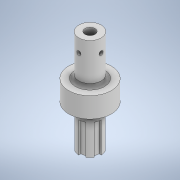
# Autodesk Inventor part: shaft
Saved by Autodesk Inventor 2020.3 (Build 243373000, 373)
## iProperties
Created: 2020-08-08
Part Number: shaft
Material: Generic
Document SubType Name: Modeling
Designer: joesp
Density: 1 g/cm^3
Appearance: Default
Author: joesp
Autodesk Inventor part; units mm, degrees
ref_plane "YZ Plane" through (0, 0, 0) normal (1, 0, 0) x (0, 1, 0)
ref_plane "XZ Plane" through (0, 0, 0) normal (0, 1, 0) x (-1, 0, 0)
ref_plane "XY Plane" through (0, 0, 0) normal (0, 0, 1) x (1, 0, 0)
sketch "Sketch1" plane through (0, 0, 0) normal (1, 0, 0) x (0, 1, 0)
  line L0 (0, 0) -> (100, 0)
  line L1 (100, 0) -> (100, -11)
  line L2 (100, -11) -> (0, -11)
  line L3 (0, -11) -> (0, 0)
  line L4 (60, -11) -> (40, -11)
  line L5 (40, -11) -> (40, -21)
  line L6 (40, -21) -> (60, -21)
  line L7 (60, -21) -> (60, -11)
  line L8 (0, -11) -> (100, -11)
  line L9 (100, -11) -> (100, -5)
  line L10 (100, -5) -> (0, -5)
  line L11 (0, -5) -> (0, -11)
  circle A0 centre (39, -12) radius 2.5
  line L12 (37.2322, -10.2322) -> (40.7678, -13.7678) construction
  circle A1 centre (61, -12) radius 2.5
  line L13 (62.7678, -10.2322) -> (59.2322, -13.7678) construction
  point P0 (0, -5)
  point P1 (60, -14.2913)
  point P2 (63.2913, -11)
  point P3 (36.7087, -11)
  point P4 (40, -14.2913)
  dimension "d1" = 11
  dimension "d2" = 100
  dimension "d3" = 10
  dimension "d4" = 20
  dimension "d5" = 40
  dimension "d7" = 6
  dimension "d31" = 5
  dimension "d32" = 45
  dimension "d33" = 1
  dimension "d34" = 1
  dimension "d35" = 5
  dimension "d36" = 45
  dimension "d37" = 1
  dimension "d38" = 1
  constraints: 28 end point, 6 parallel, 4 point on circle, 3 horizontal, 3 perpendicular, 2 centre point, 2 midpoint, 2 point on line, 1 coincident
  measures "d1" distance of L0.end L1.end
  measures "d2" distance of L0.start L0.end
  measures "d3" distance of L6.end L4.start
  measures "d4" distance of L5.end L6.end
  measures "d5" distance between parallel lines of L1 L7
  measures "d7" distance between parallel lines of L2 L10
  measures "d31" diameter of A0
  measures "d32" angle of L2 L12
  measures "d33" distance from line of L5 A0.centre
  measures "d34" distance from line of L2 A0.centre
  measures "d35" diameter of A1
  measures "d36" angle of L7 L13
  measures "d37" horizontal distance of L4.start A1.centre
  measures "d38" horizontal distance of L4.start A1.centre
revolve "Revolution1" add sketch "Sketch1" angle 360 about axis through (0, 0, 0) along (0, 1, 0) contours L10 L1 L2 A1 A0 L3 | L2 A1 L7 L6 L5 A0
sketch "Sketch2" plane through (0, 0, 0) normal (1, 0, 0) x (0, 1, 0)
  circle A0 centre (87, 0) radius 2
  line L0 (100, 11) -> (100, -11) projected
  point P0 (0, 0)
  dimension "d8" = 4
  dimension "d9" = 13
  constraints: 1 centre point
  measures "d8" diameter of A0
  measures "d9" distance from line of L0 A0.centre
extrude "Extrusion1" cut sketch "Sketch2" along normal through all both and the other way through all
sketch "Sketch3" plane through (0, 0, 0) normal (0, 0, 1) x (1, 0, 0)
  circle A0 centre (0, 87) radius 2
  line L0 (-11, 100) -> (11, 100) projected
  point P0 (0, 0)
  dimension "d12" = 13
  dimension "d13" = 4
  constraints: 1 centre point, 1 vertical alignment
  measures "d12" distance from line of L0 A0.centre
  measures "d13" diameter of A0
extrude "Extrusion2" cut sketch "Sketch3" against normal through all both and the other way through all
sketch "Sketch4" plane through (0, 0, 0) normal (0, -1, 0) x (1, 0, 0)
  circle A0 centre (0, 0) radius 9
  line L0 (-9, 0) -> (-11, 0)
  circle A1 centre (0, 0) radius 11 projected
  line L1 (0, 9) -> (0, 11)
  line L2 (9, 0) -> (11, 0)
  line L3 (0, -9) -> (0, -11)
  line L4 (-4.5, -7.7942) -> (-5.5, -9.5263)
  line L5 (-7.7942, -4.5) -> (-9.5263, -5.5)
  line L6 (-7.7942, 4.5) -> (-9.5263, 5.5)
  line L7 (-4.5, 7.7942) -> (-5.5, 9.5263)
  line L8 (4.5, 7.7942) -> (5.5, 9.5263)
  line L9 (7.7942, 4.5) -> (9.5263, 5.5)
  line L10 (7.7942, -4.5) -> (9.5263, -5.5)
  line L11 (4.5, -7.7942) -> (5.5, -9.5263)
  dimension "d21" = 18
  dimension "d22" = 30
  dimension "d23" = 30
  dimension "d24" = 30
  dimension "d25" = 30
  constraints: 24 end point, 5 perpendicular, 4 point on line, 2 horizontal, 1 coincident, 1 vertical, 35 other
  measures "d22" angle of L3 L11
  measures "d23" angle of L10 L11
  measures "d24" angle of L5 L4
  measures "d25" angle of L0 L6
extrude "Extrusion3" cut sketch "Sketch4" against normal blind 30 contours A0 L9 A1 L2 | L10 A1 L11 A0 | A0 L1 A1 L8 | L3 A1 L4 A0 | A0 L6 A1 L7 | L5 A1 L0 A0
equation "\"d34\" = d33"
equation "\"d38\" = d37"
equation "\"d23\" = d22"
equation "\"d24\" = d22"
equation "\"d25\" = d22"
body "Solid1"
